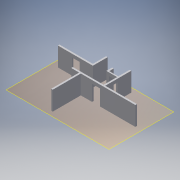
# Autodesk Inventor part: Wände_unten
Saved by Autodesk Inventor 2017 (Build 210142000, 142)
## iProperties
Created: 2017-06-01
Part Number: Wände_unten
Material: Generic
Document SubType Name: Modeling
Designer: Fake
Density: 1 g/cm^3
Appearance: Weiß
Author: Fake
Autodesk Inventor part; units mm, degrees
ref_plane "YZ Plane" through (0, 0, 0) normal (1, 0, 0) x (0, 1, 0)
ref_plane "XZ Plane" through (0, 0, 0) normal (0, 1, 0) x (-1, 0, 0)
ref_plane "Arbeitsebene1" through (0, 0, 1400) normal (0, 0, 1) x (1, 0, 0)
sketch "Skizze1" plane through (0, 0, 1400) normal (0, 0, 1) x (1, 0, 0)
  line L0 (5480, 3375) -> (5480, -3375) projected
  line L1 (5480, -3375) -> (-4000, -3375) projected
  line L2 (-4000, -3375) -> (-4000, -2075) projected
  line L3 (-4000, -2075) -> (-5480, -2075) projected
  line L4 (-5480, -2075) -> (-5480, 3375) projected
  line L5 (-5480, 3375) -> (5480, 3375) projected
  line L6 (-5480, -3575) -> (-5480, -2275) projected
  line L7 (-5480, -2275) -> (-4200, -2275) projected
  line L8 (-4200, -2275) -> (-4200, -3575) projected
  line L9 (-4200, -3575) -> (5680, -3575) projected
  line L10 (5680, -3575) -> (5680, 3575) projected
  line L11 (5680, 3575) -> (-5680, 3575) projected
  line L12 (-5680, 3575) -> (-5680, -3575) projected
  line L13 (-5680, -3575) -> (-5480, -3575) projected
  line L14 (-1140, -3375) -> (-1340, -3375)
  line L15 (-1340, -3375) -> (-1340, 25)
  line L16 (-1140, 25) -> (-1140, -3375)
  line L17 (-2310, 25) -> (-2310, 225)
  line L18 (5480, 225) -> (5480, 25)
  line L19 (-5480, 1775) -> (-1430, 1775)
  line L20 (-1230, 1575) -> (-5480, 1575)
  line L21 (-5480, 1575) -> (-5480, 1775)
  line L22 (-1230, 1575) -> (-1230, 3375)
  line L23 (-1430, 3375) -> (-1430, 1775)
  line L24 (1430, 3375) -> (1630, 3375)
  line L25 (1630, 3375) -> (1630, 225)
  line L26 (1430, 225) -> (1430, 3375)
  line L27 (5480, 25) -> (-1140, 25)
  line L28 (-1340, 25) -> (-2310, 25)
  line L29 (-2310, 225) -> (1430, 225)
  line L30 (1630, 225) -> (5480, 225)
  line L31 (-1430, 3375) -> (-1230, 3375)
  line L32 (1430, 1855) -> (130, 1855)
  line L33 (130, 1855) -> (130, 2555)
  line L34 (130, 2555) -> (330, 2555)
  line L35 (330, 2555) -> (330, 2005)
  line L36 (330, 2005) -> (1430, 2005)
  dimension "d0" = 6620
  dimension "d1" = 200
  dimension "d3" = 970
  dimension "d5" = 3850
  dimension "d6" = 3400
  dimension "d7" = 200
  dimension "d8" = 200
  dimension "d9" = 1600
  dimension "d10" = 200
  dimension "d11" = 200
  dimension "d12" = 4050
  dimension "d35" = 1630
  dimension "d36" = 200
  dimension "d37" = 150
  dimension "d38" = 700
  dimension "d40" = 1300
  constraints: 46 end point, 9 parallel, 8 perpendicular, 7 point on line, 6 horizontal, 4 collinear
  measures "d0" distance between parallel lines of L0 L16
  measures "d1" distance between parallel lines of L15 L16
  measures "d3" distance between parallel lines of L17 L15
  measures "d5" distance between parallel lines of L0 L25
  measures "d6" distance between parallel lines of L1 L27
  measures "d7" distance between parallel lines of L27 L29
  measures "d8" distance between parallel lines of L25 L26
  measures "d9" distance between parallel lines of L19 L5
  measures "d10" distance between parallel lines of L19 L20
  measures "d11" distance between parallel lines of L23 L22
  measures "d12" distance between parallel lines of L23 L4
  measures "d35" distance between parallel lines of L29 L32
  measures "d36" distance between parallel lines of L33 L35
  measures "d37" distance between parallel lines of L36 L32
  measures "d38" distance of L32.end L33.end
  measures "d40" distance between parallel lines of L26 L33
ref_plane "Arbeitsebene2" through (-5680, -3575, 3700) normal (0, 0, 1) x (1, 0, 0)
extrude "Extrusion1" add sketch "Skizze1" along normal up to surface (2300 mm away) contours L0 L27 L16 L1 L15 L28 L17 L29 L26 L5 L25 L30 | L22 L20 L4 L19 L23 L5 | L26 L32 L33 L34 L35 L36
sketch "Skizze2" plane through (-5480, 1575, 1400) normal (0, -1, 0) x (1, 0, 0)
  line L0 (4250, 2300) -> (0, 2300) projected
  line L1 (0, 0) -> (0, 2300) projected
  line L2 (0, 0) -> (4250, 0) projected
  line L3 (4250, 0) -> (4250, 2300) projected
  line L4 (4050, 0) -> (0, 0) projected
  line L5 (1700, 0) -> (2650, 0)
  line L6 (2650, 0) -> (2650, 1900)
  line L7 (2650, 1900) -> (1700, 1900)
  line L8 (1700, 1900) -> (1700, 0)
  dimension "d15" = 950
  dimension "d16" = 1600
  dimension "d17" = 1900
  constraints: 8 end point, 2 parallel, 1 horizontal, 1 perpendicular, 1 point on line
  measures "d15" distance of L6.end L7.end
  measures "d16" distance between parallel lines of L6 L3
  measures "d17" distance of L7.end L5.start
extrude "Extrusion2" cut sketch "Skizze2" against normal blind 879.25 contours L8 L7 L6 L2
sketch "Skizze3" plane through (1430, 225, 1400) normal (-1, 0, 0) x (0, 0, 1)
  line L0 (2300, 1780) -> (2300, 3150) projected
  line L1 (0, 3150) -> (2300, 3150) projected
  line L2 (0, 3150) -> (0, 1780) projected
  line L3 (0, 0) -> (2300, 0) projected
  line L4 (0, 1520) -> (1900, 1520)
  line L5 (1900, 1520) -> (1900, 570)
  line L6 (1900, 570) -> (0, 570)
  line L7 (0, 570) -> (0, 1520)
  line L8 (0, 1780) -> (2300, 1780) projected
  line L9 (0, 1630) -> (2300, 1630) projected
  line L10 (0, 1630) -> (0, 0) projected
  line L11 (2300, 0) -> (2300, 1630) projected
  dimension "d20" = 1900
  dimension "d21" = 950
  dimension "d41" = 570
  constraints: 8 end point, 2 parallel, 1 horizontal, 1 perpendicular, 1 point on line
  measures "d20" distance between parallel lines of L2 L5
  measures "d21" distance between parallel lines of L6 L4
  measures "d41" distance between parallel lines of L6 L3
extrude "Extrusion3" cut sketch "Skizze3" against normal blind 879.25 contours L7 L4 L5 L6
sketch "Skizze4" plane through (-2310, 225, 1400) normal (0, 1, 0) x (1, 0, 0)
  line L0 (0, -2300) -> (3740, -2300) projected
  line L1 (3740, 0) -> (3740, -2300) projected
  line L2 (3740, 0) -> (0, 0) projected
  line L3 (0, 0) -> (0, -2300) projected
  line L4 (3740, 0) -> (0, 0) projected
  line L5 (3480, 0) -> (2530, 0)
  line L6 (2530, 0) -> (2530, -1900)
  line L7 (2530, -1900) -> (3480, -1900)
  line L8 (3480, -1900) -> (3480, 0)
  line L9 (1170, 0) -> (1170, -2300) projected
  line L10 (1170, 0) -> (1170, -2300) projected
  dimension "d25" = 1900
  dimension "d26" = 950
  dimension "d30" = 1360
  constraints: 8 end point, 2 parallel, 1 horizontal, 1 perpendicular, 1 point on line
  measures "d25" distance between parallel lines of L2 L7
  measures "d26" distance between parallel lines of L6 L8
  measures "d30" distance between parallel lines of L9 L6
extrude "Extrusion4" cut sketch "Skizze4" against normal blind 879.25 contours L2 L8 L7 L6
sketch "Skizze5" plane through (130, 1855, 3700) normal (0, -1, 0) x (1, 0, 0)
  line L0 (1300, 0) -> (0, 0) projected
  line L1 (0, -2300) -> (0, 0) projected
  line L2 (0, -2300) -> (1300, -2300) projected
  line L3 (1300, -2300) -> (1300, 0) projected
  line L4 (0, -2300) -> (1300, -2300) projected
  line L5 (308.688, -2300) -> (1258.688, -2300)
  line L6 (1258.688, -2300) -> (1258.688, -400)
  line L7 (1258.688, -400) -> (308.688, -400)
  line L8 (308.688, -400) -> (308.688, -2300)
  dimension "d31" = 950
  dimension "d32" = 1900
  constraints: 8 end point, 2 parallel, 1 horizontal, 1 perpendicular, 1 point on line
  measures "d31" distance of L6.end L7.end
  measures "d32" distance of L7.end L5.start
extrude "Extrusion5" cut sketch "Skizze5" against normal up to surface (150 mm away) contours L2 L8 L7 L6
